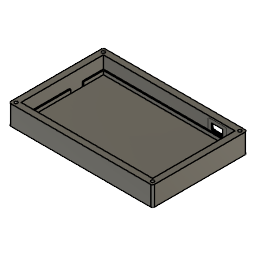
pablo_macro_case (Autodesk Fusion 360 design; units mm, degrees)
part number: 2026-03-05-21-04-07-708
Autodesk Fusion 360 part; units mm, degrees
sketch "Sketch1" plane through (0, 0, 0) normal (0, 0, 1) x (1, 0, 0)
  line L0 (-65, 50) -> (42, 50)
  line L1 (42, 50) -> (42, -17)
  line L2 (42, -17) -> (-65, -17)
  line L3 (-65, -17) -> (-65, 50)
  line L4 (-64, 49) -> (41, 49)
  line L5 (41, 49) -> (41, -16)
  line L6 (41, -16) -> (-64, -16)
  line L7 (-64, -16) -> (-64, 49)
  line L8 (-70, 55) -> (47, 55)
  line L9 (47, 55) -> (47, -22)
  line L10 (47, -22) -> (-70, -22)
  line L11 (-70, -22) -> (-70, 55)
  circle A0 centre (-67, 52) radius 1.3
  circle A1 centre (-67, -19) radius 1.3
  circle A2 centre (44, -19) radius 1.3
  circle A3 centre (44, 52) radius 1.3
  line L12 (-65, 33) -> (-64, 33)
  line L13 (-64, 33) -> (-64, 22.5)
  line L14 (-64, 22.5) -> (-65, 22.5)
  line L15 (-65, 22.5) -> (-65, 33)
  line L16 (18.5, 47.1) -> (36.3, 47.1)
  line L17 (36.3, 47.1) -> (36.3, 26.1)
  line L18 (36.3, 26.1) -> (18.5, 26.1)
  line L19 (18.5, 26.1) -> (18.5, 47.1)
  line L20 (22.9, 58) -> (31.9, 58)
  line L21 (31.9, 58) -> (31.9, 38)
  line L22 (31.9, 38) -> (22.9, 38)
  line L23 (22.9, 38) -> (22.9, 58)
  dimension "d1" = 107
  dimension "d2" = 67
  dimension "d3" = 105
  dimension "d4" = 65
  dimension "d5" = 1
  dimension "d6" = 1
  dimension "d7" = 117
  dimension "d8" = 77
  dimension "d9" = 5
  dimension "d10" = 5
  dimension "d11" = 2.6
  dimension "d12" = 2.6
  dimension "d13" = 2.6
  dimension "d14" = 2.6
  dimension "d15" = 3
  dimension "d16" = 3
  dimension "d17" = 3
  dimension "d18" = 3
  dimension "d19" = 3
  dimension "d20" = 3
  dimension "d21" = 3
  dimension "d22" = 3
  dimension "d23" = 1
  dimension "d24" = 10.5
  dimension "d25" = 17
  dimension "d26" = 17.8
  dimension "d27" = 21
  dimension "d28" = 1.9
  dimension "d29" = 4.7
  dimension "d30" = 9
  dimension "d31" = 20
  dimension "d32" = 4.4
  constraint horizontal L0
  constraint vertical L1
  constraint horizontal L2
  constraint vertical L3
  constraint horizontal L4
  constraint vertical L5
  constraint horizontal L6
  constraint vertical L7
  constraint horizontal L8
  constraint vertical L9
  constraint horizontal L10
  constraint vertical L11
  constraint horizontal L12
  constraint vertical L13
  constraint horizontal L14
  constraint vertical L15
  constraint horizontal L16
  constraint vertical L17
  constraint horizontal L18
  constraint vertical L19
  constraint horizontal L20
  constraint vertical L21
  constraint horizontal L22
  constraint vertical L23
  measures "d1" distance of L0.start L0.end
  measures "d2" distance of L0.start L2.end
  measures "d3" distance of L4.start L4.end
  measures "d4" distance of L4.start L6.end
  measures "d5" distance of L0 L4
  measures "d6" distance of L3 L7
  measures "d7" distance of L8.start L8.end
  measures "d8" distance of L8.start L10.end
  measures "d9" distance of L0 L8
  measures "d10" distance of L3 L11
  measures "d11" diameter of A0
  measures "d12" diameter of A1
  measures "d13" diameter of A2
  measures "d14" diameter of A3
  measures "d15" distance of L8 A0.centre
  measures "d16" distance of L11 A0.centre
  measures "d17" distance of L11 A1.centre
  measures "d18" distance of L10 A1.centre
  measures "d19" distance of L9 A2.centre
  measures "d20" distance of L10 A2.centre
  measures "d21" distance of L8 A3.centre
  measures "d22" distance of L9 A3.centre
  measures "d23" distance of L12.start L12.end
  measures "d24" distance of L12.start L14.end
  measures "d25" distance of L0 L12
  measures "d26" distance of L16.start L16.end
  measures "d27" distance of L16.start L18.end
  measures "d28" distance of L4 L16
  measures "d29" distance of L5 L17
  measures "d30" distance of L20.start L20.end
  measures "d31" distance of L20.start L22.end
  measures "d32" distance of L17 L21
extrude "Extrude1" add sketch "Sketch1" along normal blind 3 contours L0 L1 L2 L3 L8 L9 L10 L11 L15 L21 L23 | L0 L3 L4 L7 L12 L23 | L0 L8 L21 L23 | L0 L4 L21 L23 | L0 L1 L2 L3 L4 L5 L6 L7 L14 L21 | L4 L5 L6 L7 L13 L16 L17 L18 L19 L21 L23 | L4 L16 L21 L23 | L16 L17 L18 L19 L21 L22 L23 | L16 L21 L22 L23
extrude "Extrude2" add sketch "Sketch1" along normal blind 5 contours L0 L3 L4 L7 L12 L23 | L0 L4 L21 L23 | L0 L1 L2 L3 L4 L5 L6 L7 L14 L21
extrude "Extrude3" add 1 faces at (6, -16.6667, 5) along direction (0, 0, 1) blind 1
extrude "Extrude4" add 1 faces at (-68.3333, 18.5, 3) along direction (0, 0, 1) blind 13
extrude "Extrude5" cut sketch "Sketch1" along normal blind 12 contours L0 L8 L21 L23
extrude "Extrude6" add sketch "Sketch1" along normal blind 7 contours L0 L8 L21 L23
sketch "Sketch2" plane through (0, 55, 0) normal (0, 1, 0) x (-1, 0, 0)
  line L0 (-31.9, 7) -> (-31.9, 12)
  line L1 (-31.9, 12) -> (-22.9, 12)
  line L2 (-22.9, 12) -> (-22.9, 7)
  line L3 (-22.9, 7) -> (-31.9, 7)
  line L4 (-47, 0) -> (70, 0)
  line L5 (70, 0) -> (70, 16)
  line L6 (70, 16) -> (-47, 16)
  line L7 (-47, 16) -> (-47, 0)
  line L8 (-34.9, 14.5) -> (-19.9, 14.5)
  line L9 (-19.9, 14.5) -> (-19.9, 4.5)
  line L10 (-19.9, 4.5) -> (-34.9, 4.5)
  line L11 (-34.9, 4.5) -> (-34.9, 14.5)
  dimension "d45" = 15
  dimension "d46" = 10
  dimension "d47" = 3
  dimension "d48" = 2.5
  constraint horizontal L8
  constraint vertical L9
  constraint horizontal L10
  constraint vertical L11
  measures "d45" distance of L8.start L8.end
  measures "d46" distance of L8.start L10.end
  measures "d47" distance of L2 L9
  measures "d48" distance of L1 L8
extrude "Extrude7" cut sketch "Sketch2" against normal blind 4.5 contours L8 L9 L10 L11
fillet "Fillet1" radius 1 4 edges at (19.9, 52.75, 4.5) (34.9, 52.75, 4.5) (34.9, 52.75, 14.5) (19.9, 52.75, 14.5)
fillet "Fillet2" radius 1 8 edges at (20.1929, 55, 4.7929) (27.4, 55, 4.5) (34.6071, 55, 4.7929) (34.9, 55, 9.5) (34.6071, 55, 14.2071) (27.4, 55, 14.5) (20.1929, 55, 14.2071) (19.9, 55, 9.5)
extrude "Extrude8" add sketch "Sketch1" along normal blind 10 contours A0 | A1 | A2 | A3
fillet "Fillet3" radius 1.5 4 edges at (47, -22, 8) (47, 55, 8) (-70, 55, 8) (-70, -22, 8)
